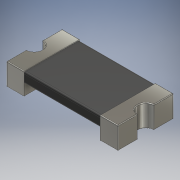
# Autodesk Inventor part: 23-12m0
Saved by Autodesk Inventor 2018 (Build 220112000, 112)
## iProperties
Created: 2019-09-26
Part Number: 23-12m0
Material: Copper
Document SubType Name: Modeling
Designer: Bradley
Density: 8.94 g/cm^3
Appearance: Smooth - Black
Author: Bradley
Autodesk Inventor part; units mm, degrees
ref_plane "YZ Plane" through (0, 0, 0) normal (1, 0, 0) x (0, 1, 0)
ref_plane "XZ Plane" through (0, 0, 0) normal (0, 1, 0) x (-1, 0, 0)
ref_plane "XY Plane" through (0, 0, 0) normal (0, 0, 1) x (1, 0, 0)
sketch "Sketch1" plane through (0, 0, 0) normal (0, 0, 1) x (1, 0, 0)
  line L0 (-1.092, -0.795) -> (1.092, -0.795)
  line L1 (1.092, -0.795) -> (1.092, 0.795)
  line L2 (1.092, 0.795) -> (-1.092, 0.795)
  line L3 (-1.092, 0.795) -> (-1.092, -0.795)
  line L4 (-1.092, -0.795) -> (1.092, 0.795) construction
  line L5 (1.092, -0.795) -> (-1.092, 0.795) construction
  line L6 (-1.092, 0.795) -> (-1.092, 0.8)
  line L7 (-1.092, 0.8) -> (-1.6, 0.8)
  line L8 (-1.6, 0.8) -> (-1.6, 0.2285)
  arc A0 (-1.6, -0.2285) -> (-1.6, 0.2285) centre (-1.6, 0) ccw
  line L9 (-1.6, -0.2285) -> (-1.6, -0.8)
  line L10 (-1.6, -0.8) -> (-1.092, -0.8)
  line L11 (-1.092, -0.8) -> (-1.092, -0.795)
  line L12 (1.092, -0.795) -> (1.092, -0.8)
  line L13 (1.092, -0.8) -> (1.6, -0.8)
  line L14 (1.6, -0.8) -> (1.6, -0.2285)
  arc A1 (1.6, 0.2285) -> (1.6, -0.2285) centre (1.6, 0) ccw
  line L15 (1.6, 0.2285) -> (1.6, 0.8)
  line L16 (1.092, 0.8) -> (1.6, 0.8)
  line L17 (1.092, 0.8) -> (1.092, 0.795)
  point P0 (0, 0)
  dimension "d0" = 3.2
  dimension "d1" = 1.6
  dimension "d2" = 1.59
  dimension "d3" = 0.508
  dimension "d4" = 0.457
  constraints: 36 end point, 12 point on line, 8 perpendicular, 5 equal length, 4 point on circle, 3 parallel, 2 centre point, 2 midpoint, 1 horizontal, 1 vertical
  measures "d0" distance between parallel lines of L15 L8
  measures "d1" distance between parallel lines of L13 L16
  measures "d2" distance between parallel lines of L0 L2
  measures "d3" distance of L16.start L15.end
  measures "d4" distance of L14.end L15.start
extrude "Extrusion1" add sketch "Sketch1" along normal blind 0.3 contours L3 L2 L1 L0
extrude "Extrusion2" add sketch "Sketch1" along normal mid plane 0.635 contours L11 L10 L9 A0 L8 L7 L6 L3 | L1 L17 L16 L15 A1 L14 L13 L12
fillet "Fillet1" radius 0.05 4 edges at (0, -0.795, 0.3) (0, -0.795, 0) (0, 0.795, 0.3) (0, 0.795, 0)
fillet "Fillet2" radius 0.02 29 edges at (-1.346, 0.8, 0.3175) (-1.6, 0.8, 0) (-1.6, 0.5142, 0.3175) (-1.6, 0.2285, 0) (-1.6, 0.5142, -0.3175) (-1.346, 0.8, -0.3175) (-1.346, -0.8, 0.3175) (-1.6, -0.5143, 0.3175) (-1.3715, 0, 0.3175) (-1.3715, 0, -0.3175) (-1.6, -0.2285, 0) (-1.6, -0.5143, -0.3175) (-1.6, -0.8, 0) (-1.346, -0.8, -0.3175) (1.346, -0.8, 0.3175) (1.6, -0.5143, 0.3175) (1.6, -0.8, 0) (1.346, -0.8, -0.3175) (1.092, 0.8, 0) (1.346, 0.8, 0.3175) (1.6, 0.5142, 0.3175) (1.3715, 0, 0.3175) (1.6, -0.2285, 0) (1.6, -0.5143, -0.3175) (1.3715, 0, -0.3175) (1.6, 0.2285, 0) (1.6, 0.5142, -0.3175) (1.346, 0.8, -0.3175) (1.6, 0.8, 0)
body "Solid1"
